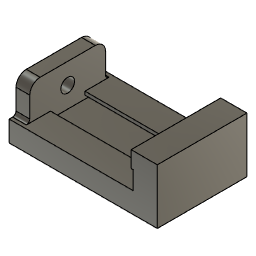
Part I - Sider v1 (Autodesk Fusion 360 design; units mm, degrees)
Autodesk Fusion 360 part; units mm, degrees
sketch "Sketch1" plane through (0, 0, 0) normal (0, 1, 0) x (1, 0, 0)
  line L0 (0, 0) -> (215, 0)
  line L1 (215, 0) -> (215, -30)
  line L2 (215, -30) -> (0, -30)
  line L3 (0, -30) -> (0, 0)
  line L4 (215, 0) -> (180, 0)
  line L5 (180, 0) -> (180, -80)
  line L6 (180, -80) -> (215, -80)
  line L7 (215, -80) -> (215, 0)
  line L8 (180, -80) -> (177, -80)
  line L9 (177, -80) -> (177, -56.3222)
  line L10 (177, -56.3222) -> (180, -56.3222)
  line L11 (180, -56.3222) -> (180, -80)
  dimension "d1" = 215
  dimension "d2" = 30
  dimension "d3" = 35
  dimension "d4" = 80
  dimension "d21" = 3
  dimension "d22" = 23.6778
  constraint horizontal L0
  constraint vertical L1
  constraint horizontal L2
  constraint vertical L3
  constraint coincident L0.start L3.end
  constraint horizontal L4
  constraint vertical L5
  constraint horizontal L6
  constraint vertical L7
  constraint horizontal L8
  constraint vertical L9
  constraint horizontal L10
  constraint vertical L11
  measures "d1" distance of L0.start L0.end
  measures "d2" distance of L0.start L2.end
  measures "d3" distance of L0.end L4.end
  measures "d4" distance of L0.end L6.end
  measures "d21" distance of L5.end L8.end
  measures "d22" distance of L5.end L10.end
extrude "Extrude1" add sketch "Sketch1" along normal blind 130 contours L0 L2 L3 L5 | L0 L1 L2 L4 L5 L7 | L2 L5 L6 L7 L11
sketch "Sketch2" plane through (0, 0, 0) normal (-1, 0, 0) x (0, -1, 0)
  line L0 (0, 0) -> (0, 30)
  line L1 (0, 30) -> (-130, 30)
  line L2 (-130, 30) -> (-130, 0)
  line L3 (-130, 0) -> (0, 0)
  line L4 (-10, 35) -> (-10, 65)
  line L5 (-25, 80) -> (-105, 80)
  line L6 (-120, 65) -> (-120, 35)
  line L7 (0, 80) -> (-130, 80)
  arc A0 (-105, 80) -> (-120, 65) centre (-105, 65) ccw
  arc A1 (-10, 65) -> (-25, 80) centre (-25, 65) ccw
  line L8 (-130, 30) -> (-125, 30)
  line L9 (-5, 30) -> (0, 30)
  arc A2 (-125, 30) -> (-120, 35) centre (-125, 35) ccw
  arc A3 (-10, 35) -> (-5, 30) centre (-5, 35) ccw
  circle A4 centre (-65, 50) radius 10
  line L10 (-105, 20) -> (-25, 20)
  line L11 (-105, 20) -> (-90, 25)
  line L12 (-40, 25) -> (-25, 20)
  line L13 (-90, 25) -> (-90, 30)
  line L14 (-40, 25) -> (-40, 30)
  point P0 (-10, 80)
  point P1 (-120, 80)
  dimension "d7" = 110
  dimension "d8" = 15
  dimension "d9" = 5
  dimension "d10" = 20
  dimension "d13" = 80
  dimension "d14" = 5
  dimension "d15" = 5
  dimension "d16" = 25
  dimension "d17" = 50
  constraint vertical L4
  constraint horizontal L5
  constraint vertical L6
  constraint coincident P0 L7
  constraint coincident L5 L7
  constraint coincident P1 L5
  constraint coincident P1 L6
  constraint tangent L5 A0
  constraint tangent L6 A0
  constraint coincident P0 L4
  constraint tangent L4 A1
  constraint tangent L5 A1
  constraint equal A0 A1
  constraint coincident L1.end L2.start
  constraint coincident L0.end L1.start
  constraint collinear L8 L9
  constraint tangent L6 A2
  constraint tangent L8 A2
  constraint tangent L4 A3
  constraint tangent L9 A3
  constraint equal A2 A3
  constraint horizontal L10
  constraint equal L11 L12
  constraint horizontal L11.end L12.start
  constraint vertical L13
  constraint perpendicular L10 L14
  constraint horizontal L13.end L14.end
  constraint horizontal L9.start L14.end
  measures "d7" distance of P0 P1
  measures "d8" radius of A0
  measures "d9" radius of A2
  measures "d10" diameter of A4
  measures "d13" distance of L10.start L10.end
  measures "d14" distance of L12.start L14.end
  measures "d15" distance of L10 L12.start
  measures "d16" horizontal distance of L0.start L10.end
  measures "d17" distance of L13 L14
extrude "Extrude2" add sketch "Sketch2" against normal blind 20 contours L1 L4 L5 L6 L7 A0 A1 A2 A3
extrude "Extrude3" cut sketch "Sketch2" against normal up to surface (160 mm away) from surface at -20 contours L1 L10 L11 L12 L13 L14
extrude "Extrude4" add sketch "Sketch1" along normal blind 130 contours L5 L8 L9 L10 L11
